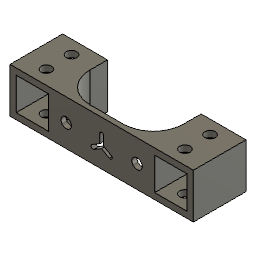
MountingBracket-Alternate (Autodesk Fusion 360 design; units mm, degrees)
Autodesk Fusion 360 part; units mm, degrees
sketch "Sketch1" plane through (0, 0, 0) normal (0, 0, 1) x (1, 0, 0)
  line L0 (7.1, 7.1) -> (-7.1, 7.1)
  line L1 (-7.1, 7.1) -> (-7.1, -7.1)
  line L2 (-7.1, -7.1) -> (7.1, -7.1)
  line L3 (7.1, -7.1) -> (7.1, 7.1)
  line L4 (0, 3) -> (0, -1) construction
  line L5 (-0.75, 3) -> (-0.75, -1)
  line L6 (0.75, 3) -> (0.75, -1)
  circle A0 centre (0, 3) radius 0.75
  line L7 (-3.0891, -3.6495) -> (0.375, -1.6495)
  circle A1 centre (-3.4641, -3) radius 0.75
  line L8 (-3.8391, -2.3505) -> (-0.375, -0.3505)
  line L9 (-3.4641, -3) -> (0, -1) construction
  line L10 (3.8391, -2.3505) -> (0.375, -0.3505)
  circle A2 centre (3.4641, -3) radius 0.75
  line L11 (3.0891, -3.6495) -> (-0.375, -1.6495)
  line L12 (3.4641, -3) -> (0, -1) construction
  line L13 (-4.2141, 3.75) -> (4.2141, 3.75)
  line L14 (4.2141, 3.75) -> (4.2141, -3.75)
  line L15 (4.2141, -3.75) -> (-4.2141, -3.75)
  line L16 (-4.2141, -3.75) -> (-4.2141, 3.75)
  line L17 (-7.1, 0) -> (7.1, 0) construction
  line L18 (0, 7.1) -> (0, -7.1) construction
  point P0 (0, -3.75)
  point P1 (-4.2141, 0)
  dimension "d38" = 14.2
  dimension "d41" = 4
  dimension "d42" = 0.75
  dimension "d43" = -0.75
  dimension "d45" = 360
  constraint horizontal L0
  constraint perpendicular L0 L1
  constraint parallel L0 L2
  constraint parallel L1 L3
  constraint equal L0 L3
  constraint vertical L4
  constraint coincident L6.start A0
  constraint tangent L6 A0
  constraint coincident L5.start A0
  constraint coincident L4.start A0.centre
  constraint equal L4 L5
  constraint equal L4 L6
  constraint horizontal L13
  constraint vertical L14
  constraint horizontal L15
  constraint vertical L16
  constraint tangent A0 L13
  constraint tangent A1 L16
  constraint tangent A2 L14
  constraint tangent A2 L15
  constraint midpoint L15 P0
  constraint midpoint L16 P1
  constraint midpoint L1 L17.start
  constraint midpoint L3 L17.end
  constraint midpoint L0 L18.start
  constraint midpoint L2 L18.end
  constraint coincident origin L18
  constraint coincident origin L17
  constraint coincident P0 L18
  constraint coincident P1 L17
  measures "d38" distance of L0.start L2.end
  measures "d41" distance of L4.start L4.end
extrude "Extrude1" add sketch "Sketch1" along normal blind 2 contours L0 L1 L2 L3 | L5 A0 A1 L8 L13 L16 | L6 A0 L10 A2 L13 L14 | A1 L15 L16 | A2 L14 L15 | L7 A1 A2 L11 L15
sketch "Sketch2" plane through (0, 0, 0) normal (0, 0, 1) x (1, 0, 0)
  line L0 (-33.9, 6.35) -> (-21.2, 6.35) construction
  line L1 (-21.2, 6.35) -> (-21.2, -6.35) construction
  line L2 (-21.2, -6.35) -> (-33.9, -6.35) construction
  line L3 (-33.9, -6.35) -> (-33.9, 6.35) construction
  line L4 (21.2, 6.35) -> (33.9, 6.35) construction
  line L5 (33.9, 6.35) -> (33.9, -6.35) construction
  line L6 (33.9, -6.35) -> (21.2, -6.35) construction
  line L7 (21.2, -6.35) -> (21.2, 6.35) construction
  line L8 (-21.2, 0) -> (21.2, 0) construction
  line L9 (-21.1, -6.45) -> (-34, -6.45)
  line L10 (-34, -6.45) -> (-34, 6.45)
  line L11 (-34, 6.45) -> (-21.1, 6.45)
  line L12 (-21.1, 6.45) -> (-21.1, -6.45)
  line L13 (-18.6, -8.95) -> (-36.5, -8.95)
  line L14 (-36.5, -8.95) -> (-36.5, 8.95)
  line L15 (-36.5, 8.95) -> (-18.6, 8.95)
  line L16 (-18.6, 8.95) -> (-18.6, -8.95)
  line L17 (0, 2.5) -> (0, 20)
  line L18 (34, -6.45) -> (34, 6.45)
  line L19 (34, 6.45) -> (21.1, 6.45)
  line L20 (21.1, 6.45) -> (21.1, -6.45)
  line L21 (21.1, -6.45) -> (34, -6.45)
  line L22 (36.5, -8.95) -> (36.5, 8.95)
  line L23 (36.5, 8.95) -> (18.6, 8.95)
  line L24 (18.6, -8.95) -> (36.5, -8.95)
  line L25 (18.6, 8.95) -> (18.6, -8.95)
  line L26 (-18.6, -2.6) -> (-18.6, -8.95)
  line L27 (-18.6, 8.95) -> (18.6, 8.95)
  line L28 (18.6, -8.95) -> (-18.6, -8.95)
  line L29 (-7.1, 7.1) -> (-7.1, -7.1)
  line L30 (-7.1, -7.1) -> (7.1, -7.1)
  line L31 (7.1, -7.1) -> (7.1, 7.1)
  line L32 (7.1, 7.1) -> (-7.1, 7.1)
  dimension "d18" = 12.7
  dimension "d19" = 12.7
  dimension "d20" = 42.4
  dimension "d23" = -2.5
  constraint horizontal L0
  constraint vertical L1
  constraint horizontal L2
  constraint vertical L3
  constraint horizontal L4
  constraint vertical L5
  constraint horizontal L6
  constraint vertical L7
  constraint equal L0 L4
  constraint equal L3 L7
  constraint collinear L0 L4
  constraint midpoint L1 L8.start
  constraint midpoint L7 L8.end
  constraint coincident L8 origin
  constraint midpoint L8 origin
  constraint symmetric L9.start L17 L20.end
  constraint symmetric L9.end L17 L18.start
  constraint symmetric L10.end L17 L18.end
  constraint symmetric L11.end L17 L19.end
  constraint symmetric L13.start L17 L24.start
  constraint symmetric L13.end L17 L22.start
  constraint symmetric L14.end L17 L22.end
  constraint symmetric L15.end L17 L23.end
  constraint vertical L26
  measures "d18" distance of L0.start L0.end
  measures "d19" distance of L0.start L2.end
  measures "d20" distance of L1 L7
extrude "Extrude2" add sketch "Sketch2" along normal blind 2
extrude "Extrude3" add sketch "Sketch2" against normal blind 19 contours L13 L14 L15 L16 L26 | L22 L23 L24 L25
fillet "Fillet1" radius 12 2 edges at (-18.6, 0, 0) (18.6, 0, 0)
sketch "Sketch3" plane through (0, 8.95, 0) normal (0, 1, 0) x (-1, 0, 0)
  line L0 (36.5, -19) -> (36.5, 2)
  line L1 (36.5, 2) -> (-36.5, 2)
  line L2 (18.6, -12) -> (18.6, -19)
  line L3 (-36.5, -19) -> (-18.6, -19)
  circle A0 centre (-27.55, -13.6) radius 2.075
  circle A1 centre (-27.55, -3.6) radius 2.075
  line L4 (-27.55, -19) -> (-27.55, 2) construction
  line L5 (-36.5, 2) -> (-36.5, -19)
  line L6 (-18.6, -19) -> (-18.6, -12)
  line L7 (18.6, -19) -> (36.5, -19)
  line L8 (0, 1.75) -> (0, 22.5)
  circle A2 centre (27.55, -13.6) radius 2.075
  circle A3 centre (27.55, -3.6) radius 2.075
  dimension "d32" = 4.15
  dimension "d33" = 10
  dimension "d34" = 5.6
  constraint equal A0 A1
  constraint midpoint L3 L4.start
  constraint coincident A0.centre L4
  constraint coincident A1.centre L4
  constraint coincident L1 L4.end
  constraint vertical L4
  constraint symmetric A0 L8 A2
  constraint symmetric A1 L8 A3
  measures "d32" diameter of A0
  measures "d33" distance of A0.centre A1.centre
  measures "d34" distance of L1 A1.centre
extrude "Extrude4" cut sketch "Sketch3" against normal blind 17.9
sketch "Sketch4" plane through (0, 0, 2) normal (0, 0, 1) x (1, 0, 0)
  line L0 (36.5, -8.95) -> (36.5, 8.95)
  line L1 (36.5, 8.95) -> (-36.5, 8.95)
  line L2 (-36.5, 8.95) -> (-36.5, -8.95)
  line L3 (-36.5, -8.95) -> (36.5, -8.95)
  line L4 (-34, 6.45) -> (-21.1, 6.45)
  line L5 (-21.1, 6.45) -> (-21.1, -6.45)
  line L6 (-21.1, -6.45) -> (-34, -6.45)
  line L7 (-34, -6.45) -> (-34, 6.45)
  line L8 (34, -6.45) -> (21.1, -6.45)
  line L9 (21.1, -6.45) -> (21.1, 6.45)
  line L10 (21.1, 6.45) -> (34, 6.45)
  line L11 (34, 6.45) -> (34, -6.45)
  line L12 (0.75, -0.567) -> (3.8391, -2.3505)
  arc A0 (3.0891, -3.6495) -> (3.8391, -2.3505) centre (3.4641, -3) ccw
  line L13 (3.0891, -3.6495) -> (0, -1.866)
  line L14 (0, -1.866) -> (-3.0891, -3.6495)
  arc A1 (-3.8391, -2.3505) -> (-3.0891, -3.6495) centre (-3.4641, -3) ccw
  line L15 (-3.8391, -2.3505) -> (-0.75, -0.567)
  line L16 (-0.75, -0.567) -> (-0.75, 3)
  arc A2 (0.75, 3) -> (-0.75, 3) centre (0, 3) ccw
  line L17 (0.75, 3) -> (0.75, -0.567)
  line L18 (21.1, -6.45) -> (21.1, 6.45)
  line L19 (-21.1, 6.45) -> (-21.1, -6.45)
  circle A3 centre (-14.1, 0) radius 2.075
  line L20 (-21.1, 0) -> (21.1, 0) construction
  line L21 (0, 2.5) -> (0, 20)
  circle A4 centre (14.1, 0) radius 2.075
  dimension "d47" = 4.15
  dimension "d48" = 7
  constraint midpoint L19 L20.start
  constraint midpoint L9 L20.end
  constraint coincident A3.centre L20
  constraint symmetric A3 L21 A4
  measures "d47" diameter of A3
  measures "d48" distance of L5 A3.centre
extrude "Extrude5" cut sketch "Sketch4" against normal blind 21 contours A3 | A4
ref_plane "WorkPlane1" through (0, 0, -8) normal (0, 0, -1) x (-1, 0, 0)
sketch "Sketch5" plane through (0, 0, -8) normal (0, 0, -1) x (-1, 0, 0)
  line L0 (-21.1, 6.45) -> (-21.1, -6.45)
  line L1 (21.1, -6.45) -> (21.1, 6.45)
  line L2 (-21.1, 0) -> (21.1, 0) construction
  circle A0 centre (-14.1, 0) radius 4.5
  line L3 (-17.7, 2.7) -> (-17.7, -2.7)
  line L4 (0, 1.75) -> (0, 22.5)
  circle A1 centre (14.1, 0) radius 4.5
  line L5 (17.7, 2.7) -> (17.7, -2.7)
  dimension "d52" = 9
  dimension "d53" = 7
  dimension "d54" = 3.6
  constraint midpoint L0 L2.start
  constraint midpoint L1 L2.end
  constraint coincident L2 A0.centre
  constraint coincident A0 L3.start
  constraint coincident A0 L3.end
  constraint vertical L3
  constraint symmetric A0 L4 A1
  constraint symmetric L3.start L4 L5.start
  constraint symmetric L3.end L4 L5.end
  measures "d52" diameter of A0
  measures "d53" distance of L0 A0.centre
  measures "d54" distance of A0.centre L3
extrude "Extrude6" cut sketch "Sketch5" against normal blind 8 contours A0 L3 | A1 L5 picked at (-15.0162, 0.2196) picked at (14.4429, 0.1257)
equation "mounting_size = 1.5 mm"
equation "d16 = frontal_width"
equation "d21 = -tolerance_bar"
equation "tolerance_bar = 0.1 mm"
equation "d25 = frontal_width"
equation "d30 = 13 mm - ( 4 / 4 ) * 1 mm"
equation "tolerance_hole = 0.15 mm"
equation "d32 = 4 mm + tolerance_hole"
equation "d42 = mounting_size / 2"
equation "d43 = -d42"
equation "frontal_width = 2 mm"
equation "d47 = 4 mm + tolerance_hole"
